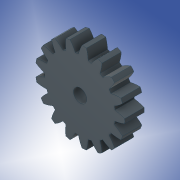
# Autodesk Inventor part: Motor Gear
Saved by Autodesk Inventor 2017 SP1 (Build 210196100, 196)
## iProperties
Created: 2017-07-05
Part Number: Motor Gear
Material: ABS Plastic
Document SubType Name: Modeling
Designer: zallen
Density: 1.06 g/cm^3
Appearance: CR Dark Blue
Author: zallen
Autodesk Inventor part; units mm, degrees
ref_plane "YZ Plane" through (0, 0, 0) normal (1, 0, 0) x (0, 1, 0)
ref_plane "XZ Plane" through (0, 0, 0) normal (0, 1, 0) x (-1, 0, 0)
ref_plane "XY Plane" through (0, 0, 0) normal (0, 0, 1) x (1, 0, 0)
sketch "Sketch1" plane through (0, 0, 0) normal (0, 0, 1) x (1, 0, 0)
  circle A0 centre (0, 0) radius 14.5
  line L0 (0, 0) -> (16, 0) construction
  arc A1 (18.3614, 0.9) -> (14.3614, 2) centre (12.4223, -12.8741) ccw
  arc A2 (14.3614, -2) -> (18.3614, -0.9) centre (12.4223, 12.8741) ccw
  arc A3 (14.3614, -2) -> (14.3614, 2) centre (0, 0) ccw
  arc A4 (18.3614, -0.9) -> (18.3614, 0.9) centre (-1.6183, 0) ccw
  arc A5 (16.7964, 7.4721) -> (12.6691, 7.0529) centre (16.2341, -7.5173) ccw
  arc A6 (17.4466, 5.7937) -> (16.7964, 7.4721) centre (-1.5091, -0.5846) ccw
  arc A7 (14.1141, 3.323) -> (17.4466, 5.7937) centre (6.9328, 16.4922) ccw
  arc A8 (14.1141, 3.323) -> (12.6691, 7.0529) centre (0, 0) ccw
  arc A9 (12.9629, 13.0351) -> (9.2658, 11.1532) centre (17.8534, -1.1453) ccw
  arc A10 (14.1756, 11.7049) -> (12.9629, 13.0351) centre (-1.196, -1.0903) ccw
  arc A11 (11.9606, 8.1972) -> (14.1756, 11.7049) centre (0.5069, 17.8829) ccw
  arc A12 (11.9606, 8.1972) -> (9.2658, 11.1532) centre (0, 0) ccw
  arc A13 (7.3787, 16.8376) -> (4.6111, 13.7473) centre (17.0615, 5.3815) ccw
  arc A14 (8.99, 16.0353) -> (7.3787, 16.8376) centre (-0.7214, -1.4487) ccw
  arc A15 (8.1918, 11.9643) -> (8.99, 16.0353) centre (-5.9874, 16.8585) ccw
  arc A16 (8.1918, 11.9643) -> (4.6111, 13.7473) centre (0, 0) ccw
  arc A17 (0.798, 18.3661) -> (-0.6664, 14.4847) centre (13.9654, 11.1814) ccw
  arc A18 (2.5903, 18.2) -> (0.798, 18.3661) centre (-0.1493, -1.6114) ccw
  arc A19 (3.3166, 14.1156) -> (2.5903, 18.2) centre (-11.673, 13.5572) ccw
  arc A20 (3.3166, 14.1156) -> (-0.6664, 14.4847) centre (0, 0) ccw
  arc A21 (-5.8905, 17.4142) -> (-5.8538, 13.2658) centre (8.9832, 15.4712) ccw
  arc A22 (-4.1592, 17.9068) -> (-5.8905, 17.4142) centre (0.4429, -1.5566) ccw
  arc A23 (-2.0065, 14.3605) -> (-4.1592, 17.9068) centre (-15.7822, 8.4249) ccw
  arc A24 (-2.0065, 14.3605) -> (-5.8538, 13.2658) centre (0, 0) ccw
  arc A25 (-11.7834, 14.1103) -> (-10.2507, 10.2554) centre (2.7877, 17.6716) ccw
  arc A26 (-10.347, 15.1951) -> (-11.7834, 14.1103) centre (0.9753, -1.2915) ccw
  arc A27 (-7.0586, 12.6659) -> (-10.347, 15.1951) centre (-17.7599, 2.1548) ccw
  arc A28 (-7.0586, 12.6659) -> (-10.2507, 10.2554) centre (0, 0) ccw
  arc A29 (-16.085, 8.9008) -> (-13.2632, 5.8599) centre (-3.7843, 17.4853) ccw
  arc A30 (-15.1374, 10.4312) -> (-16.085, 8.9008) centre (1.3759, -0.8519) ccw
  arc A31 (-11.1574, 9.2607) -> (-15.1374, 10.4312) centre (-17.339, -4.4063) ccw
  arc A32 (-11.1574, 9.2607) -> (-13.2632, 5.8599) centre (0, 0) ccw
  arc A33 (-18.2141, 2.4892) -> (-14.4844, 0.673) centre (-9.8451, 14.9375) ccw
  arc A34 (-17.8834, 4.2586) -> (-18.2141, 2.4892) centre (1.5908, -0.2974) ccw
  arc A35 (-13.7494, 4.6048) -> (-17.8834, 4.2586) centre (-14.5764, -10.3723) ccw
  arc A36 (-13.7494, 4.6048) -> (-14.4844, 0.673) centre (0, 0) ccw
  arc A37 (-17.8834, -4.2586) -> (-13.7494, -4.6048) centre (-14.5764, 10.3723) ccw
  arc A38 (-18.2141, -2.4892) -> (-17.8834, -4.2586) centre (1.5908, 0.2974) ccw
  arc A39 (-14.4844, -0.673) -> (-18.2141, -2.4892) centre (-9.8451, -14.9375) ccw
  arc A40 (-14.4844, -0.673) -> (-13.7494, -4.6048) centre (0, 0) ccw
  arc A41 (-15.1374, -10.4312) -> (-11.1574, -9.2607) centre (-17.339, 4.4063) ccw
  arc A42 (-16.085, -8.9008) -> (-15.1374, -10.4312) centre (1.3759, 0.8519) ccw
  arc A43 (-13.2632, -5.8599) -> (-16.085, -8.9008) centre (-3.7843, -17.4853) ccw
  arc A44 (-13.2632, -5.8599) -> (-11.1574, -9.2607) centre (0, 0) ccw
  arc A45 (-10.347, -15.1951) -> (-7.0586, -12.6659) centre (-17.7599, -2.1548) ccw
  arc A46 (-11.7834, -14.1103) -> (-10.347, -15.1951) centre (0.9753, 1.2915) ccw
  arc A47 (-10.2507, -10.2554) -> (-11.7834, -14.1103) centre (2.7877, -17.6716) ccw
  arc A48 (-10.2507, -10.2554) -> (-7.0586, -12.6659) centre (0, 0) ccw
  arc A49 (-4.1592, -17.9068) -> (-2.0065, -14.3605) centre (-15.7822, -8.4249) ccw
  arc A50 (-5.8905, -17.4142) -> (-4.1592, -17.9068) centre (0.4429, 1.5566) ccw
  arc A51 (-5.8538, -13.2658) -> (-5.8905, -17.4142) centre (8.9832, -15.4712) ccw
  arc A52 (-5.8538, -13.2658) -> (-2.0065, -14.3605) centre (0, 0) ccw
  arc A53 (2.5903, -18.2) -> (3.3166, -14.1156) centre (-11.673, -13.5572) ccw
  arc A54 (0.798, -18.3661) -> (2.5903, -18.2) centre (-0.1493, 1.6114) ccw
  arc A55 (-0.6664, -14.4847) -> (0.798, -18.3661) centre (13.9654, -11.1814) ccw
  arc A56 (-0.6664, -14.4847) -> (3.3166, -14.1156) centre (0, 0) ccw
  arc A57 (8.99, -16.0353) -> (8.1918, -11.9643) centre (-5.9874, -16.8585) ccw
  arc A58 (7.3787, -16.8376) -> (8.99, -16.0353) centre (-0.7214, 1.4487) ccw
  arc A59 (4.6111, -13.7473) -> (7.3787, -16.8376) centre (17.0615, -5.3815) ccw
  arc A60 (4.6111, -13.7473) -> (8.1918, -11.9643) centre (0, 0) ccw
  arc A61 (14.1756, -11.7049) -> (11.9606, -8.1972) centre (0.5069, -17.8829) ccw
  arc A62 (12.9629, -13.0351) -> (14.1756, -11.7049) centre (-1.196, 1.0903) ccw
  arc A63 (9.2658, -11.1532) -> (12.9629, -13.0351) centre (17.8534, 1.1453) ccw
  arc A64 (9.2658, -11.1532) -> (11.9606, -8.1972) centre (0, 0) ccw
  arc A65 (17.4466, -5.7937) -> (14.1141, -3.323) centre (6.9328, -16.4922) ccw
  arc A66 (16.7964, -7.4721) -> (17.4466, -5.7937) centre (-1.5091, 0.5846) ccw
  arc A67 (12.6691, -7.0529) -> (16.7964, -7.4721) centre (16.2341, 7.5173) ccw
  arc A68 (12.6691, -7.0529) -> (14.1141, -3.323) centre (0, 0) ccw
  point P0 (18.3817, 0)
  point P1 (17.1404, 6.6402)
  point P2 (13.5842, 12.3836)
  point P3 (8.1934, 16.4546)
  point P4 (1.696, 18.3033)
  point P5 (-5.0304, 17.68)
  point P6 (-11.0774, 14.6689)
  point P7 (-15.6284, 9.6767)
  point P8 (-18.0687, 3.3776)
  point P9 (-18.0687, -3.3776)
  point P10 (-15.6284, -9.6767)
  point P11 (-11.0774, -14.6689)
  point P12 (-5.0304, -17.68)
  point P13 (1.696, -18.3033)
  point P14 (8.1934, -16.4546)
  point P15 (13.5842, -12.3836)
  point P16 (17.1404, -6.6402)
  dimension "d0" = 29
  dimension "d1" = 16
  dimension "d2" = 15
  dimension "d3" = 4
  dimension "d4" = 2
  dimension "d6" = 1.8
  dimension "d15" = 20
  dimension "d18" = 360
  constraints: 137 point on circle, 68 centre point, 3 symmetric about line, 2 end point, 1 coincident, 1 horizontal, 1 point on line, 228 other
  measures "d1" distance of L0.start L0.end
  measures "d2" radius of A1
  measures "d3" horizontal distance of A1.start A1.end
  measures "d4" distance from line of L0 A1.end
  measures "d6" distance of A2.end A1.start
  measures "d15" radius of A4
extrude "Extrusion1" add sketch "Sketch1" along normal blind 8
sketch "Sketch5" plane through (0, 0, 8) normal (0, 0, 1) x (1, 0, 0)
  circle A0 centre (0, 0) radius 2.75
  dimension "d32" = 5.5
  constraints: 1 centre point, 1 coincident
  measures "d32" diameter of A0
extrude "Extrusion5" cut sketch "Sketch5" against normal through all
body "Solid1"
